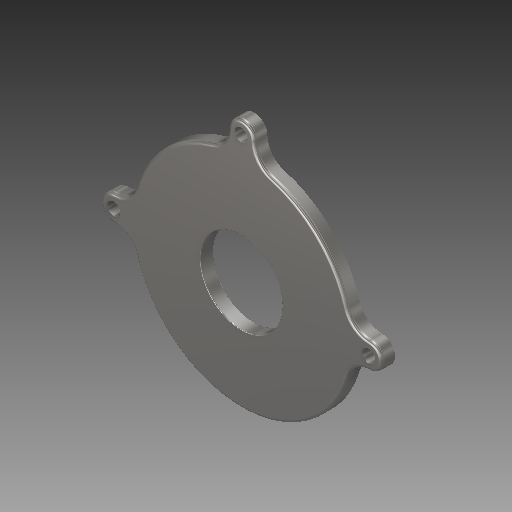
# Autodesk Inventor part: PillowCover
Saved by Autodesk Inventor 2018 (Build 220112000, 112)
## iProperties
Created: 2017-10-18
Part Number: PillowCover
Material: Steel, Mild
Document SubType Name: Modeling
Designer: Bryce Richards
Density: 7.85 g/cm^3
Appearance: Semi-Polished
Mass: 122.322 g
Surface Area: 93.4048 cm^2
Volume: 15.5825 cm^3
Author: Bryce Richards
Autodesk Inventor part; units mm, degrees
ref_plane "YZ Plane" through (0, 0, 0) normal (1, 0, 0) x (0, 1, 0)
ref_plane "XZ Plane" through (0, 0, 0) normal (0, 1, 0) x (-1, 0, 0)
ref_plane "XY Plane" through (0, 0, 0) normal (0, 0, 1) x (1, 0, 0)
sketch "Sketch1" plane through (0, 0, 0) normal (0, 0, 1) x (1, 0, 0)
  circle A0 centre (0, 10.4747) radius 26 construction
  arc A1 (2.8969, 46.7164) -> (-2.8969, 46.7164) centre (0, 49.4747) ccw construction
  circle A2 centre (0, 49.4747) radius 2 construction
  arc A3 (36.3889, 7.4445) -> (36.2417, 13.3716) centre (39, 10.4747) ccw construction
  circle A4 centre (39, 10.4747) radius 2 construction
  arc A5 (-36.2417, 13.3716) -> (-36.3889, 7.4445) centre (-39, 10.4747) ccw construction
  circle A6 centre (-39, 10.4747) radius 2 construction
  arc A7 (33.5, 10.4747) -> (-33.5, 10.4747) centre (0, 10.4747) ccw construction
  arc A8 (4, 49.4747) -> (-4, 49.4747) centre (0, 49.4747) ccw
  circle A9 centre (0, 49.4747) radius 2
  arc A10 (39, 6.4747) -> (39, 14.4747) centre (39, 10.4747) ccw
  circle A11 centre (39, 10.4747) radius 2
  circle A12 centre (-39, 10.4747) radius 2
  arc A13 (-39, 14.4747) -> (-39, 6.4747) centre (-39, 10.4747) ccw
  line L0 (-4, 49.4747) -> (-4, 49.4522)
  line L1 (4, 49.4747) -> (4, 49.4522)
  arc A14 (-9.0988, 42.7154) -> (-4, 49.4522) centre (-11, 49.4522) ccw
  arc A15 (4, 49.4522) -> (9.0988, 42.7154) centre (11, 49.4522) ccw
  line L2 (-39, 14.4747) -> (-38.9776, 14.4747)
  line L3 (-39, 6.4747) -> (-38.9776, 6.4747)
  line L4 (39, 14.4747) -> (38.9776, 14.4747)
  line L5 (39, 6.4747) -> (38.9776, 6.4747)
  arc A16 (-9.0988, 42.7154) -> (-32.2407, 19.5735) centre (0, 10.4747) ccw
  arc A17 (-32.2407, 1.3759) -> (32.2407, 1.3759) centre (0, 10.4747) ccw
  arc A18 (32.2407, 19.5735) -> (9.0988, 42.7154) centre (0, 10.4747) ccw
  arc A19 (-38.9776, 14.4747) -> (-32.2407, 19.5735) centre (-38.9776, 21.4747) ccw
  arc A20 (-32.2407, 1.3759) -> (-38.9776, 6.4747) centre (-38.9776, -0.5253) ccw
  arc A21 (38.9776, 6.4747) -> (32.2407, 1.3759) centre (38.9776, -0.5253) ccw
  arc A22 (32.2407, 19.5735) -> (38.9776, 14.4747) centre (38.9776, 21.4747) ccw
  point P0 (0, 0)
  point P1 (-33.2603, 14.4747)
  point P2 (-33.2603, 6.4747)
  point P3 (33.2603, 14.4747)
  point P4 (33.2603, 6.4747)
  dimension "d1" = 7
  dimension "d2" = 7
  dimension "d3" = 7
  dimension "d4" = 33.5
  dimension "d5" = 33.5
  dimension "d6" = 33.5
  constraints: 28 point on circle, 20 tangent, 15 centre point, 12 end point, 9 equal radius, 8 point on line, 7 coincident, 2 vertical, 1 horizontal, 1 parallel
  measures "d1" radius of A14
  measures "d2" radius of A15
  measures "d3" radius of A19
  measures "d4" radius of A18
  measures "d5" radius of A17
  measures "d6" radius of A16
extrude "Extrusion1" add sketch "Sketch1" along normal blind 4
fillet "Fillet1" radius 1 18 edges at (-34.7531, 15.8931, 4) (-38.9888, 14.4747, 4) (-43, 10.4747, 4) (-38.9888, 6.4747, 4) (-34.7531, 5.0563, 4) (0, -23.0253, 4) (34.7531, 5.0563, 4) (38.9888, 6.4747, 4) (43, 10.4747, 4) (38.9888, 14.4747, 4) (34.7531, 15.8931, 4) (23.6881, 34.1628, 4) (5.4184, 45.2278, 4) (4, 49.4635, 4) (0, 53.4747, 4) (-4, 49.4635, 4) (-5.4184, 45.2278, 4) (-23.6881, 34.1628, 4)
sketch "Sketch2" plane through (0, 0, 0) normal (0, 0, -1) x (-1, 0, 0)
  circle A0 centre (0, 10.4747) radius 26 construction
  circle A1 centre (0, 10.4747) radius 26
  circle A2 centre (0, 10.4747) radius 22.5
  point P0 (0, 0)
  dimension "d12" = 45
  constraints: 2 centre point, 2 coincident, 1 concentric
  measures "d12" diameter of A2
extrude "Extrusion2" add sketch "Sketch2" along normal blind 5
sketch "Sketch3" plane through (0, 0, 4) normal (0, 0, 1) x (1, 0, 0)
  circle A0 centre (0, 10.4747) radius 12.5 construction
  circle A1 centre (0, 10.4747) radius 12.5
  point P0 (0, 0)
  constraints: 1 centre point, 1 coincident, 1 concentric
extrude "Extrusion3" cut sketch "Sketch3" against normal up to next
fillet "Fillet2" radius 0.25 2 edges at (-12.5, 10.4747, 0) (-12.5, 10.4747, 4)
body "Solid1"
